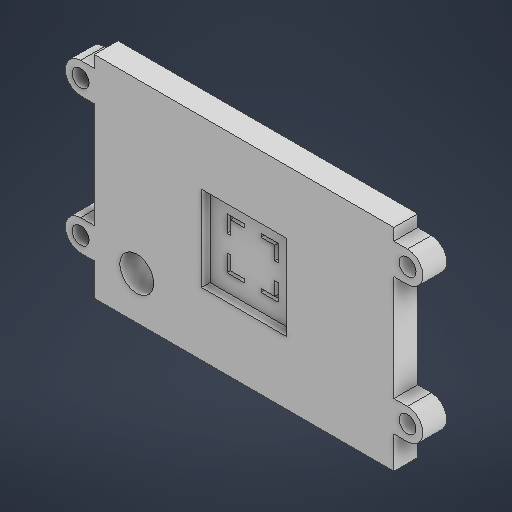
# Autodesk Inventor part: soporte p2
Saved by Autodesk Inventor 2026.1 (Build 301233020, 233B)
## iProperties
Created: 2026-01-16
Part Number: soporte p2
Material: Generic
Document SubType Name: Modeling
Designer: Marcelo
Density: 1 g/cm^3
Appearance: Default
Mass: 37.9424 g
Surface Area: 145.351 cm^2
Volume: 37.9424 cm^3
Author: Marcelo
Autodesk Inventor part; units mm, degrees
ref_plane "YZ Plane" through (0, 0, 0) normal (1, 0, 0) x (0, 1, 0)
ref_plane "XZ Plane" through (0, 0, 0) normal (0, 1, 0) x (-1, 0, 0)
ref_plane "XY Plane" through (0, 0, 0) normal (0, 0, 1) x (1, 0, 0)
sketch "Sketch1" plane through (0, 0, 0) normal (0, 0, 1) x (1, 0, 0)
  line L0 (44, -31) -> (-44, -31)
  line L1 (-44, -31) -> (-44, 31)
  line L2 (-44, 31) -> (44, 31)
  line L3 (44, 31) -> (44, -31)
  line L4 (44, -31) -> (-44, 31) construction
  line L5 (-44, -31) -> (44, 31) construction
  point P0 (0, 0)
  dimension "d0" = 88
  dimension "d1" = 62
  constraints: 12 end point, 2 midpoint, 2 parallel, 1 horizontal, 1 perpendicular
  measures "d0" distance of L1.end L2.end
  measures "d1" distance of L0.end L1.end
extrude "Extrusion1" add sketch "Sketch1" along normal blind 7
sketch "Sketch2" plane through (0, 0, 7) normal (0, 0, 1) x (1, 0, 0)
  circle A0 centre (-48, 23) radius 2.5
  line L0 (-48, 23) -> (-44, 23)
  line L1 (-44, 31) -> (-44, -31) projected
  arc A1 (-48, 27.5) -> (-48, 18.5) centre (-48, 23) ccw
  line L2 (44, 31) -> (-44, 31) projected
  line L3 (-44, 29.1847) -> (-44, 31)
  line L4 (-44, 16.8153) -> (-44, 18.5)
  line L5 (0, 54.4598) -> (0, -54.4598) construction
  circle A2 centre (48, 23) radius 2.5
  line L6 (48, 23) -> (44, 23)
  line L7 (44, 31) -> (44, -31)
  arc A3 (48, 18.5) -> (48, 27.5) centre (48, 23) ccw
  line L8 (44, 29.1847) -> (44, 31)
  line L9 (44, 16.8153) -> (44, 18.5)
  circle A4 centre (48, -17) radius 2.5
  line L10 (48, -17) -> (44, -17)
  arc A5 (48, -21.5) -> (48, -12.5) centre (48, -17) ccw
  line L11 (44, -10.8153) -> (44, -9)
  line L12 (44, -23.1847) -> (44, -21.5)
  line L13 (-44, 29.1847) -> (-44, 31)
  line L14 (-44, 16.8153) -> (-44, -9)
  line L15 (-44, -23.1847) -> (-44, -31)
  line L16 (44, 29.1847) -> (44, 31)
  line L17 (44, 16.8153) -> (44, -10.8153)
  line L18 (44, -31) -> (44, 31) projected
  line L19 (44, -23.1847) -> (44, -31)
  line L20 (44, 18.5) -> (48, 18.5)
  line L21 (44, 27.5) -> (48, 27.5)
  line L22 (44, -21.5) -> (48, -21.5)
  line L23 (44, -12.5) -> (48, -12.5)
  line L24 (-48, 27.5) -> (-44, 27.5)
  line L25 (-48, 27.5) -> (-44, 27.5) construction
  line L26 (-48, 18.5) -> (-44, 18.5)
  line L27 (-44, -17) -> (-48, -17)
  circle A6 centre (-48, -17) radius 2.5
  arc A7 (-48, -12.5) -> (-48, -21.5) centre (-48, -17) ccw
  line L28 (-48, -21.5) -> (-44, -21.5)
  line L29 (-48, -12.5) -> (-44, -12.5)
  point P0 (0, 0)
  point P1 (-44, 20.9384)
  point P2 (-44, 25.0616)
  point P3 (-46.6154, 27.2817)
  point P4 (-46.6154, 18.7183)
  point P5 (44, 20.9384)
  point P6 (44, 25.0616)
  point P7 (46.6154, 27.2817)
  point P8 (46.6154, 18.7183)
  point P9 (46.6154, -12.7183)
  point P10 (46.6954, -21.4151)
  point P11 (44, -19.0616)
  point P12 (44, -14.9384)
  point P13 (44, -23.1847)
  dimension "d4" = 5
  dimension "d5" = 4
  dimension "d6" = 2
  dimension "d32" = 8
  dimension "d43" = 4
  dimension "d44" = 5
  dimension "d45" = 2
  dimension "d46" = 40
  dimension "d47" = 0
  dimension "d48" = 5
  dimension "d49" = 2
  dimension "d50" = 40
  dimension "d51" = 4
  constraints: 52 end point, 14 point on circle, 12 symmetric about line, 9 horizontal, 8 centre point, 8 point on line, 8 tangent, 7 vertical, 2 collinear, 1 coincident, 1 midpoint, 1 perpendicular, 22 other
  measures "d4" diameter of A0
  measures "d5" distance of L0.start L0.end
  measures "d6" radial gap between concentric circles of A0 A1
  measures "d32" distance between parallel lines of L2 L6
  measures "d43" distance of L10.start L10.end
  measures "d44" diameter of A4
  measures "d45" radial gap between concentric circles of A4 A5
  measures "d46" distance between parallel lines of L6 L10
  measures "d47" distance between parallel lines of L24 L25
  measures "d48" diameter of A6
  measures "d49" radial gap between concentric circles of A6 A7
  measures "d50" distance between parallel lines of L0 L27
  measures "d51" distance of L27.start L27.end
extrude "Extrusion2" add sketch "Sketch2" against normal blind 7
sketch "Sketch3" plane through (0, 0, 7) normal (0, 0, 1) x (1, 0, 0)
  line L0 (12.5, -12.5) -> (-12.5, -12.5)
  line L1 (-12.5, -12.5) -> (-12.5, 12.5)
  line L2 (-12.5, 12.5) -> (12.5, 12.5)
  line L3 (12.5, 12.5) -> (12.5, -12.5)
  line L4 (12.5, -12.5) -> (-12.5, 12.5) construction
  line L5 (-12.5, -12.5) -> (12.5, 12.5) construction
  point P0 (0, 0)
  dimension "d33" = 25
  dimension "d34" = 25
  constraints: 12 end point, 2 midpoint, 2 parallel, 1 horizontal, 1 perpendicular
  measures "d33" distance of L1.end L2.end
  measures "d34" distance of L0.end L1.end
extrude "Extrusion3" cut sketch "Sketch3" against normal blind 2.5
sketch "Sketch4" plane through (0, 0, 4.5) normal (0, 0, 1) x (1, 0, 0)
  line L0 (-12.5, 12.5) -> (12.5, 12.5) projected
  line L1 (-12.5, -12.5) -> (-12.5, 12.5) projected
  line L2 (12.5, -12.5) -> (-12.5, -12.5) projected
  line L3 (12.5, 12.5) -> (12.5, -12.5) projected
  line L4 (7.5, 7.5) -> (-7.5, 7.5)
  line L5 (-7.5, 7.5) -> (-7.5, -7.5)
  line L6 (-7.5, -7.5) -> (7.5, -7.5)
  line L7 (7.5, -7.5) -> (7.5, 7.5)
  line L8 (-6.5, 6.5) -> (6.5, 6.5)
  line L9 (6.5, 6.5) -> (6.5, -6.5)
  line L10 (6.5, -6.5) -> (-6.5, -6.5)
  line L11 (-6.5, -6.5) -> (-6.5, 6.5)
  line L12 (-9.9797, 2.5) -> (9.6006, 2.5)
  line L13 (-9.9797, -2.5) -> (9.6006, -2.5)
  line L14 (-2.5, 9.6233) -> (-2.5, -10.0692)
  line L15 (2.5, 9.6233) -> (2.5, -9.2277)
  point P0 (0, 0)
  point P1 (-2.5, -7.5)
  point P2 (-2.5, -6.5)
  point P3 (-6.5, -2.5)
  point P4 (-7.5, -2.5)
  point P5 (2.5, -6.5)
  point P6 (2.5, -7.5)
  point P7 (7.5, -2.5)
  point P8 (6.5, -2.5)
  point P9 (2.5, 7.5)
  point P10 (2.5, 6.5)
  point P11 (6.5, 2.5)
  point P12 (7.5, 2.5)
  point P13 (-2.5, 6.5)
  point P14 (-2.5, 7.5)
  point P15 (-7.5, 2.5)
  point P16 (-6.5, 2.5)
  dimension "d35" = 5
  dimension "d36" = 1
  dimension "d37" = 5
  dimension "d38" = 5
  dimension "d39" = 5
  dimension "d40" = 5
  constraints: 24 end point, 3 perpendicular, 1 horizontal, 6 other
  measures "d35" distance between parallel lines of L0 L4
  measures "d36" distance between parallel lines of L4 L8
  measures "d37" distance between parallel lines of L7 L15
  measures "d38" distance between parallel lines of L5 L14
  measures "d39" distance between parallel lines of L6 L13
  measures "d40" distance between parallel lines of L4 L12
extrude "Extrusion4" cut sketch "Sketch4" against normal blind 1 contours L7 L12 L9 L8 L15 L4 | L14 L8 L11 L12 L5 L4 | L7 L6 L15 L10 L9 L13 | L13 L11 L10 L14 L6 L5
sketch "Sketch5" plane through (0, 0, 0) normal (0, 0, -1) x (-1, 0, 0)
  circle A0 centre (31.5, -18.5) radius 5
  line L0 (44, -21.5) -> (44, -31) projected
  line L1 (44, -31) -> (-44, -31) projected
  point P0 (0, 0)
  dimension "d52" = 10
  dimension "d53" = 12.5
  dimension "d54" = 12.5
  constraints: 1 centre point
  measures "d52" diameter of A0
  measures "d53" distance from line of L0 A0.centre
  measures "d54" distance from line of L1 A0.centre
extrude "Extrusion5" cut sketch "Sketch5" against normal blind 7
body "Solid1"
